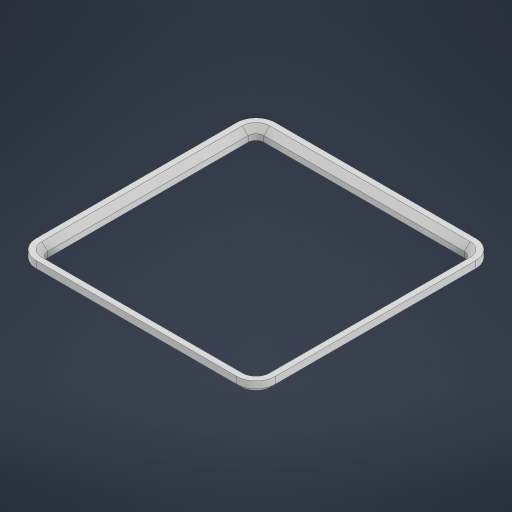
# Autodesk Inventor part: top_insert
Saved by Autodesk Inventor 2024 (Build 280153000, 153)
## iProperties
Created: 2024-03-20
Part Number: top_insert
Material: Všeobecné
Document SubType Name: Modeling
Designer: Simak
Density: 1 g/cm^3
Appearance: Výchozí
Author: Simak
Autodesk Inventor part; units mm, degrees
ref_plane "YZ Plane" through (0, 0, 0) normal (1, 0, 0) x (0, 1, 0)
ref_plane "XZ Plane" through (0, 0, 0) normal (0, 1, 0) x (-1, 0, 0)
ref_plane "XY Plane" through (0, 0, 0) normal (0, 0, 1) x (1, 0, 0)
sketch "Náčrt1" plane through (0, 0, 0) normal (0, 1, 0) x (-1, 0, 0)
  line L0 (50, -44) -> (50, 44)
  line L1 (44, 50) -> (-44, 50)
  line L2 (-50, 44) -> (-50, -44)
  line L3 (-44, -50) -> (44, -50)
  line L4 (50, 50) -> (0, 0) construction
  line L5 (0, 0) -> (-50, -50) construction
  line L6 (0, 0) -> (-50, 50) construction
  arc A0 (44, -50) -> (50, -44) centre (44, -44) ccw
  arc A1 (-50, -44) -> (-44, -50) centre (-44, -44) ccw
  arc A2 (-44, 50) -> (-50, 44) centre (-44, 44) ccw
  arc A3 (50, 44) -> (44, 50) centre (44, 44) ccw
  point P0 (50, -50)
  dimension "d0" = 100
  dimension "d1" = 100
  dimension "d2" = 6
  constraints: 14 end point, 8 point on circle, 8 point on line, 8 tangent, 4 centre point, 3 equal radius, 2 horizontal, 2 perpendicular, 2 vertical
  measures "d0" distance of L6.end L5.end
  measures "d1" distance of L5.end point (50, -50)
  measures "d2" radius of A0
sketch "Náčrt2" plane through (0, 0, 0) normal (0, 0, 1) x (1, 0, 0)
  line L0 (47.5, -2.5) -> (52.5, -2.5)
  line L1 (52.5, -2.5) -> (52.5, 2.5)
  line L2 (52.5, 2.5) -> (50, 2.5)
  line L3 (50, 2.5) -> (47.5, 0)
  line L4 (47.5, 0) -> (47.5, -2.5)
  line L5 (52.5, -0.5) -> (50.5, -2.5)
  point P0 (0, 0)
  point P1 (50, 0)
  point P2 (50, 0)
  point P3 (50, 0)
  dimension "d3" = 2.5
  dimension "d4" = 2.5
  dimension "d5" = 5
  dimension "d8" = 2
  constraints: 12 end point, 3 perpendicular, 2 parallel, 2 point on line, 1 horizontal, 1 horizontal alignment, 1 vertical alignment
  measures "d3" distance from line of L1 point (50, 0)
  measures "d4" distance from line of point (50, 0) L0
  measures "d5" distance of L0.end L1.end
  measures "d8" distance from line of L0 L5.start
sweep "Tažení1" add profiles "Náčrt2" path "Náčrt1" path curves L2 A2 L1 A3 L0 A0 L3 A1 contours L4 L3 L2 L1 L5 L0
equation "\"d1\" = d0"
